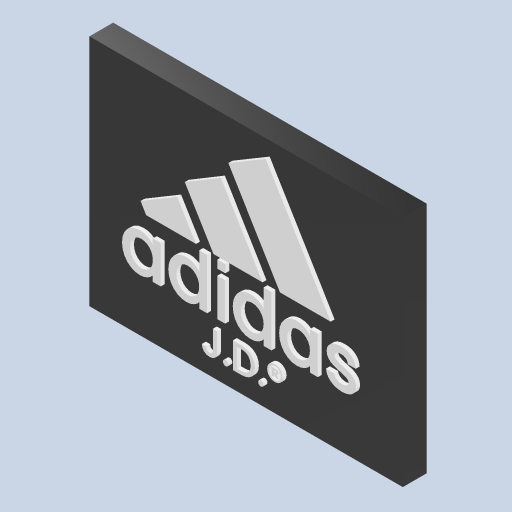
# Autodesk Inventor part: Logo1
Saved by Autodesk Inventor 2023 (Build 270158000, 158)
## iProperties
Created: 2024-02-26
Part Number: Logo1
Material: Generic
Document SubType Name: Modeling
Designer: dsone
Density: 1 g/cm^3
Appearance: Default
Author: dsone
Autodesk Inventor part; units mm, degrees
ref_plane "YZ Plane" through (0, 0, 0) normal (1, 0, 0) x (0, 1, 0)
ref_plane "XZ Plane" through (0, 0, 0) normal (0, 1, 0) x (-1, 0, 0)
ref_plane "XY Plane" through (0, 0, 0) normal (0, 0, 1) x (1, 0, 0)
sketch "Sketch1" plane through (0, 0, 0) normal (0, 0, 1) x (1, 0, 0)
  line L0 (0, 0) -> (240, 0)
  line L1 (240, 0) -> (240, 137)
  line L2 (240, 137) -> (0, 137)
  line L3 (0, 137) -> (0, 0)
  line L4 (0, 0) -> (0, 12)
  line L5 (240, 137) -> (209, 137)
  line L6 (0, 137) -> (10, 137)
  line L7 (0, 137) -> (72, 137)
  line L8 (0, 137) -> (94, 137)
  line L9 (0, 137) -> (158, 137)
  line L10 (0, 137) -> (183, 137)
  line L11 (0, 0) -> (0, 27)
  line L12 (0, 0) -> (0, 43)
  line L13 (0, 0) -> (0, 116)
  line L14 (0, 0) -> (7, 0)
  line L15 (0, 0) -> (70, 0)
  line L16 (0, 0) -> (92, 0)
  line L17 (0, 0) -> (154, 0)
  line L18 (0, 0) -> (176, 0)
  line L19 (7, 0) -> (0, 12)
  line L20 (70, 0) -> (46.1151, 39.5808)
  line L21 (92, 0) -> (55.7734, 60.525)
  line L22 (154, 0) -> (101.369, 87.9322)
  line L23 (176, 0) -> (110.8056, 108.9223)
  line L24 (240, 0) -> (158, 137)
  line L25 (110.8056, 108.9223) -> (158, 137)
  line L26 (0, 12) -> (46.1151, 39.5808)
  line L27 (55.7734, 60.525) -> (101.369, 87.9322)
  line L28 (-19.7944, -2.3315) -> (269.4882, -2.3315) construction
  line L29 (269.4882, -2.3315) -> (269.4882, -75.7518) construction
  line L30 (269.4882, -75.7518) -> (-19.7944, -75.7518) construction
  line L31 (-19.7944, -75.7518) -> (-19.7944, -2.3315) construction
  line L32 (14.2994, -81.6937) -> (242.7128, -81.6937) construction
  line L33 (242.7128, -81.6937) -> (242.7128, -137.0896) construction
  line L34 (242.7128, -137.0896) -> (14.2994, -137.0896) construction
  line L35 (14.2994, -137.0896) -> (14.2994, -81.6937) construction
  spline S0 degree 2 poles (-23.4452, -44.8067) (-23.4452, -37.678) (-17.5046, -26.6137) (-7.2571, -20.4503) (-1.0194, -20.4503) knots 0 0 0 1 2 3 3 3
  spline S1 degree 2 poles (-1.0194, -20.4503) (4.6241, -20.4503) (12.9409, -24.9057) (15.4657, -28.1731) knots 0 0 0 1 2 2 2
  line L36 (15.4657, -28.1731) -> (15.4657, -21.2671)
  line L37 (15.4657, -21.2671) -> (25.4162, -21.2671)
  line L38 (25.4162, -21.2671) -> (25.4162, -68.7919)
  line L39 (25.4162, -68.7919) -> (15.4657, -68.7919)
  line L40 (15.4657, -68.7919) -> (15.4657, -61.7374)
  spline S2 degree 2 poles (15.4657, -61.7374) (12.9409, -65.079) (4.3271, -69.5344) (-1.168, -69.5344) knots 0 0 0 1 2 2 2
  spline S3 degree 2 poles (-1.168, -69.5344) (-7.3313, -69.5344) (-17.5046, -63.2968) (-23.4452, -51.9354) (-23.4452, -44.8067) knots 0 0 0 1 2 3 3 3
  spline S4 degree 2 poles (15.4657, -44.9552) (15.4657, -40.0542) (11.3815, -32.777) (4.8469, -28.9899) (1.0598, -28.9899) knots 0 0 0 1 2 3 3 3
  spline S5 degree 2 poles (1.0598, -28.9899) (-2.7274, -28.9899) (-9.262, -32.7028) (-13.3462, -39.9057) (-13.3462, -44.8067) knots 0 0 0 1 2 3 3 3
  spline S6 degree 2 poles (-13.3462, -44.8067) (-13.3462, -49.7077) (-9.262, -57.1335) (-2.6531, -60.9948) (1.0598, -60.9948) knots 0 0 0 1 2 3 3 3
  spline S7 degree 2 poles (1.0598, -60.9948) (4.8469, -60.9948) (11.3815, -57.2077) (15.4657, -49.9305) (15.4657, -44.9552) knots 0 0 0 1 2 3 3 3
  spline S8 degree 2 poles (35.0697, -44.8067) (35.0697, -37.678) (41.0103, -26.6137) (51.2578, -20.4503) (57.5697, -20.4503) knots 0 0 0 1 2 3 3 3
  spline S9 degree 2 poles (57.5697, -20.4503) (62.2479, -20.4503) (71.3073, -24.5344) (73.9806, -27.876) knots 0 0 0 1 2 2 2
  line L41 (73.9806, -27.876) -> (73.9806, -4.9305)
  line L42 (73.9806, -4.9305) -> (83.931, -4.9305)
  line L43 (83.931, -4.9305) -> (83.931, -68.7919)
  line L44 (83.931, -68.7919) -> (73.9806, -68.7919)
  line L45 (73.9806, -68.7919) -> (73.9806, -61.6632)
  spline S10 degree 2 poles (73.9806, -61.6632) (71.6043, -65.079) (62.9905, -69.5344) (57.4954, -69.5344) knots 0 0 0 1 2 2 2
  spline S11 degree 2 poles (57.4954, -69.5344) (51.2578, -69.5344) (41.0103, -63.2968) (35.0697, -51.9354) (35.0697, -44.8067) knots 0 0 0 1 2 3 3 3
  spline S12 degree 2 poles (73.9806, -44.9552) (73.9806, -40.0542) (69.8964, -32.777) (63.3617, -28.9899) (59.5746, -28.9899) knots 0 0 0 1 2 3 3 3
  spline S13 degree 2 poles (59.5746, -28.9899) (55.7875, -28.9899) (49.2528, -32.7028) (45.1687, -39.9057) (45.1687, -44.8067) knots 0 0 0 1 2 3 3 3
  spline S14 degree 2 poles (45.1687, -44.8067) (45.1687, -49.7077) (49.2528, -57.1335) (55.8617, -60.9948) (59.5746, -60.9948) knots 0 0 0 1 2 3 3 3
  spline S15 degree 2 poles (59.5746, -60.9948) (63.3617, -60.9948) (69.8964, -57.2077) (73.9806, -49.9305) (73.9806, -44.9552) knots 0 0 0 1 2 3 3 3
  line L46 (106.7281, -21.2671) -> (106.7281, -68.7919)
  line L47 (106.7281, -68.7919) -> (96.8518, -68.7919)
  line L48 (96.8518, -68.7919) -> (96.8518, -21.2671)
  line L49 (96.8518, -21.2671) -> (106.7281, -21.2671)
  spline S16 degree 2 poles (101.9013, -14.9552) (99.2281, -14.9552) (95.5895, -11.3166) (95.5895, -8.6434) knots 0 0 0 1 2 2 2
  spline S17 degree 2 poles (95.5895, -8.6434) (95.5895, -5.9701) (99.2281, -2.3315) (101.9013, -2.3315) knots 0 0 0 1 2 2 2
  spline S18 degree 2 poles (101.9013, -2.3315) (104.4261, -2.3315) (108.0647, -5.9701) (108.0647, -8.6434) knots 0 0 0 1 2 2 2
  spline S19 degree 2 poles (108.0647, -8.6434) (108.0647, -11.3166) (104.4261, -14.9552) (101.9013, -14.9552) knots 0 0 0 1 2 2 2
  spline S20 degree 2 poles (116.3815, -44.8067) (116.3815, -37.678) (122.3221, -26.6137) (132.5697, -20.4503) (138.8815, -20.4503) knots 0 0 0 1 2 3 3 3
  spline S21 degree 2 poles (138.8815, -20.4503) (143.5598, -20.4503) (152.6192, -24.5344) (155.2924, -27.876) knots 0 0 0 1 2 2 2
  line L50 (155.2924, -27.876) -> (155.2924, -4.9305)
  line L51 (155.2924, -4.9305) -> (165.2429, -4.9305)
  line L52 (165.2429, -4.9305) -> (165.2429, -68.7919)
  line L53 (165.2429, -68.7919) -> (155.2924, -68.7919)
  line L54 (155.2924, -68.7919) -> (155.2924, -61.6632)
  spline S22 degree 2 poles (155.2924, -61.6632) (152.9162, -65.079) (144.3023, -69.5344) (138.8073, -69.5344) knots 0 0 0 1 2 2 2
  spline S23 degree 2 poles (138.8073, -69.5344) (132.5697, -69.5344) (122.3221, -63.2968) (116.3815, -51.9354) (116.3815, -44.8067) knots 0 0 0 1 2 3 3 3
  spline S24 degree 2 poles (155.2924, -44.9552) (155.2924, -40.0542) (151.2083, -32.777) (144.6736, -28.9899) (140.8865, -28.9899) knots 0 0 0 1 2 3 3 3
  spline S25 degree 2 poles (140.8865, -28.9899) (137.0994, -28.9899) (130.5647, -32.7028) (126.4806, -39.9057) (126.4806, -44.8067) knots 0 0 0 1 2 3 3 3
  spline S26 degree 2 poles (126.4806, -44.8067) (126.4806, -49.7077) (130.5647, -57.1335) (137.1736, -60.9948) (140.8865, -60.9948) knots 0 0 0 1 2 3 3 3
  spline S27 degree 2 poles (140.8865, -60.9948) (144.6736, -60.9948) (151.2083, -57.2077) (155.2924, -49.9305) (155.2924, -44.9552) knots 0 0 0 1 2 3 3 3
  spline S28 degree 2 poles (174.8964, -44.8067) (174.8964, -37.678) (180.837, -26.6137) (191.0845, -20.4503) (197.3221, -20.4503) knots 0 0 0 1 2 3 3 3
  spline S29 degree 2 poles (197.3221, -20.4503) (202.9657, -20.4503) (211.2825, -24.9057) (213.8073, -28.1731) knots 0 0 0 1 2 2 2
  line L55 (213.8073, -28.1731) -> (213.8073, -21.2671)
  line L56 (213.8073, -21.2671) -> (223.7578, -21.2671)
  line L57 (223.7578, -21.2671) -> (223.7578, -68.7919)
  line L58 (223.7578, -68.7919) -> (213.8073, -68.7919)
  line L59 (213.8073, -68.7919) -> (213.8073, -61.7374)
  spline S30 degree 2 poles (213.8073, -61.7374) (211.2825, -65.079) (202.6687, -69.5344) (197.1736, -69.5344) knots 0 0 0 1 2 2 2
  spline S31 degree 2 poles (197.1736, -69.5344) (191.0103, -69.5344) (180.837, -63.2968) (174.8964, -51.9354) (174.8964, -44.8067) knots 0 0 0 1 2 3 3 3
  spline S32 degree 2 poles (213.8073, -44.9552) (213.8073, -40.0542) (209.7231, -32.777) (203.1885, -28.9899) (199.4013, -28.9899) knots 0 0 0 1 2 3 3 3
  spline S33 degree 2 poles (199.4013, -28.9899) (195.6142, -28.9899) (189.0796, -32.7028) (184.9954, -39.9057) (184.9954, -44.8067) knots 0 0 0 1 2 3 3 3
  spline S34 degree 2 poles (184.9954, -44.8067) (184.9954, -49.7077) (189.0796, -57.1335) (195.6885, -60.9948) (199.4013, -60.9948) knots 0 0 0 1 2 3 3 3
  spline S35 degree 2 poles (199.4013, -60.9948) (203.1885, -60.9948) (209.7231, -57.2077) (213.8073, -49.9305) (213.8073, -44.9552) knots 0 0 0 1 2 3 3 3
  spline S36 degree 2 poles (253.9806, -69.5344) (248.337, -69.5344) (239.4261, -65.5245) (234.3023, -58.5443) (234.0796, -54.2374) knots 0 0 0 1 2 3 3 3
  line L60 (234.0796, -54.2374) -> (244.2528, -54.2374)
  spline S37 degree 2 poles (244.2528, -54.2374) (244.5499, -57.2077) (249.8221, -61.2919) (253.7578, -61.2919) knots 0 0 0 1 2 2 2
  spline S38 degree 2 poles (253.7578, -61.2919) (257.9162, -61.2919) (262.5202, -58.0988) (262.5202, -55.5741) knots 0 0 0 1 2 2 2
  spline S39 degree 2 poles (262.5202, -55.5741) (262.5202, -52.9008) (257.3964, -50.3018) (251.9013, -48.7424) knots 0 0 0 1 2 2 2
  spline S40 degree 2 poles (251.9013, -48.7424) (246.5548, -47.3315) (239.7974, -44.5097) (234.8964, -38.8661) (234.8964, -34.1879) knots 0 0 0 1 2 3 3 3
  spline S41 degree 2 poles (234.8964, -34.1879) (234.8964, -30.4008) (239.3518, -24.0889) (247.7429, -20.4503) (253.1637, -20.4503) knots 0 0 0 1 2 3 3 3
  spline S42 degree 2 poles (253.1637, -20.4503) (261.2578, -20.4503) (271.2083, -28.6929) (271.5796, -35.7473) knots 0 0 0 1 2 2 2
  line L61 (271.5796, -35.7473) -> (261.7033, -35.7473)
  spline S43 degree 2 poles (261.7033, -35.7473) (261.4806, -32.5542) (256.8023, -28.7671) (252.7924, -28.7671) knots 0 0 0 1 2 2 2
  spline S44 degree 2 poles (252.7924, -28.7671) (248.931, -28.7671) (244.7726, -31.6632) (244.7726, -34.1137) knots 0 0 0 1 2 2 2
  spline S45 degree 2 poles (244.7726, -34.1137) (244.7726, -35.9701) (247.5944, -38.5691) (251.5301, -40.0542) (255.3914, -41.1681) knots 0 0 0 1 2 3 3 3
  spline S46 degree 2 poles (255.3914, -41.1681) (260.5895, -42.579) (267.2726, -45.4008) (272.0994, -50.8958) (272.1736, -55.4998) knots 0 0 0 1 2 3 3 3
  spline S47 degree 2 poles (272.1736, -55.4998) (272.1736, -59.584) (267.6439, -65.9701) (259.4756, -69.5344) (253.9806, -69.5344) knots 0 0 0 1 2 3 3 3
  line L62 (96.6197, -82.1362) -> (96.6197, -105.5933)
  spline S48 degree 2 poles (96.6197, -105.5933) (96.6197, -109.9387) (91.3087, -114.9681) (87.0035, -114.9681) knots 0 0 0 1 2 2 2
  spline S49 degree 2 poles (87.0035, -114.9681) (82.6984, -114.9681) (77.4276, -109.9387) (77.4276, -105.5933) knots 0 0 0 1 2 2 2
  line L63 (77.4276, -105.5933) -> (82.8191, -105.5933)
  spline S50 degree 2 poles (82.8191, -105.5933) (82.8593, -107.7258) (84.9515, -110.2606) (87.0035, -110.2606) knots 0 0 0 1 2 2 2
  spline S51 degree 2 poles (87.0035, -110.2606) (89.0555, -110.2606) (91.2282, -107.6856) (91.2282, -105.5933) knots 0 0 0 1 2 2 2
  line L64 (91.2282, -105.5933) -> (91.2282, -82.1362)
  line L65 (91.2282, -82.1362) -> (96.6197, -82.1362)
  spline S52 degree 2 poles (107.443, -114.9681) (105.9945, -114.9681) (104.023, -112.9966) (104.023, -111.5481) knots 0 0 0 1 2 2 2
  spline S53 degree 2 poles (104.023, -111.5481) (104.023, -110.0997) (105.9945, -108.1281) (107.443, -108.1281) knots 0 0 0 1 2 2 2
  spline S54 degree 2 poles (107.443, -108.1281) (108.811, -108.1281) (110.7825, -110.0997) (110.7825, -111.5481) knots 0 0 0 1 2 2 2
  spline S55 degree 2 poles (110.7825, -111.5481) (110.7825, -112.9966) (108.811, -114.9681) (107.443, -114.9681) knots 0 0 0 1 2 2 2
  spline S56 degree 2 poles (127.1582, -82.1362) (132.3485, -82.1362) (140.1542, -86.1195) (144.4191, -93.563) (144.4191, -98.5119) knots 0 0 0 1 2 3 3 3
  spline S57 degree 2 poles (144.4191, -98.5119) (144.4191, -103.4609) (140.1542, -110.7837) (132.3485, -114.6462) (127.1582, -114.6462) knots 0 0 0 1 2 3 3 3
  line L66 (127.1582, -114.6462) -> (116.5361, -114.6462)
  line L67 (116.5361, -114.6462) -> (116.5361, -82.1362)
  line L68 (116.5361, -82.1362) -> (127.1582, -82.1362)
  spline S58 degree 2 poles (127.1582, -110.3008) (132.8716, -110.3008) (138.9471, -104.1449) (138.9471, -98.5119) knots 0 0 0 1 2 2 2
  spline S59 degree 2 poles (138.9471, -98.5119) (138.9471, -92.879) (132.8716, -86.4816) (127.1582, -86.4816) knots 0 0 0 1 2 2 2
  line L69 (127.1582, -86.4816) -> (121.8874, -86.4816)
  line L70 (121.8874, -86.4816) -> (121.8874, -110.3008)
  line L71 (121.8874, -110.3008) -> (127.1582, -110.3008)
  spline S60 degree 2 poles (151.8626, -114.9681) (150.4141, -114.9681) (148.4426, -112.9966) (148.4426, -111.5481) knots 0 0 0 1 2 2 2
  spline S61 degree 2 poles (148.4426, -111.5481) (148.4426, -110.0997) (150.4141, -108.1281) (151.8626, -108.1281) knots 0 0 0 1 2 2 2
  spline S62 degree 2 poles (151.8626, -108.1281) (153.2306, -108.1281) (155.2021, -110.0997) (155.2021, -111.5481) knots 0 0 0 1 2 2 2
  spline S63 degree 2 poles (155.2021, -111.5481) (155.2021, -112.9966) (153.2306, -114.9681) (151.8626, -114.9681) knots 0 0 0 1 2 2 2
  spline S64 degree 2 poles (169.5661, -81.6937) (172.3825, -81.6937) (176.8084, -84.2285) (179.303, -88.6543) (179.303, -91.4708) knots 0 0 0 1 2 3 3 3
  spline S65 degree 2 poles (179.303, -91.4708) (179.303, -94.247) (176.8084, -98.7131) (172.3825, -101.2077) (169.5661, -101.2077) knots 0 0 0 1 2 3 3 3
  spline S66 degree 2 poles (169.5661, -101.2077) (166.7496, -101.2077) (162.3237, -98.7131) (159.7889, -94.247) (159.7889, -91.4708) knots 0 0 0 1 2 3 3 3
  spline S67 degree 2 poles (159.7889, -91.4708) (159.7889, -88.6543) (162.3237, -84.2285) (166.7496, -81.6937) (169.5661, -81.6937) knots 0 0 0 1 2 3 3 3
  spline S68 degree 2 poles (169.5661, -99.0752) (172.9458, -99.0752) (177.0096, -94.8505) (177.0096, -91.4708) knots 0 0 0 1 2 2 2
  spline S69 degree 2 poles (177.0096, -91.4708) (177.0096, -88.0508) (172.9458, -83.8261) (169.5661, -83.8261) knots 0 0 0 1 2 2 2
  spline S70 degree 2 poles (169.5661, -83.8261) (166.1461, -83.8261) (162.1226, -88.0508) (162.1226, -91.4708) knots 0 0 0 1 2 2 2
  spline S71 degree 2 poles (162.1226, -91.4708) (162.1226, -94.8505) (166.1461, -99.0752) (169.5661, -99.0752) knots 0 0 0 1 2 2 2
  spline S72 degree 2 poles (173.8712, -89.5797) (173.8712, -90.6259) (172.8251, -92.1548) (171.9399, -92.5169) knots 0 0 0 1 2 2 2
  line L72 (171.9399, -92.5169) -> (174.4345, -96.3795)
  line L73 (174.4345, -96.3795) -> (170.8938, -96.3795)
  line L74 (170.8938, -96.3795) -> (168.8016, -92.879)
  line L75 (168.8016, -92.879) -> (168.4797, -92.879)
  line L76 (168.4797, -92.879) -> (168.4797, -96.3795)
  line L77 (168.4797, -96.3795) -> (165.5425, -96.3795)
  line L78 (165.5425, -96.3795) -> (165.5425, -86.3207)
  line L79 (165.5425, -86.3207) -> (170.2501, -86.3207)
  spline S73 degree 2 poles (170.2501, -86.3207) (171.8997, -86.3207) (173.8712, -88.1313) (173.8712, -89.5797) knots 0 0 0 1 2 2 2
  line L80 (168.4797, -90.4649) -> (170.0891, -90.4649)
  spline S74 degree 2 poles (170.0891, -90.4649) (170.4512, -90.4649) (170.9743, -90.0626) (170.9743, -89.6602) knots 0 0 0 1 2 2 2
  spline S75 degree 2 poles (170.9743, -89.6602) (170.9743, -89.2981) (170.4512, -88.936) (170.0891, -88.936) knots 0 0 0 1 2 2 2
  line L81 (170.0891, -88.936) -> (168.4797, -88.936)
  line L82 (168.4797, -88.936) -> (168.4797, -90.4649)
  dimension "d0" = 240
  dimension "d1" = 137
  dimension "d2" = 12
  dimension "d3" = 31
  dimension "d4" = 10
  dimension "d5" = 72
  dimension "d6" = 94
  dimension "d7" = 158
  dimension "d8" = 183
  dimension "d9" = 27
  dimension "d10" = 43
  dimension "d11" = 116
  dimension "d12" = 7
  dimension "d13" = 70
  dimension "d14" = 92
  dimension "d15" = 154
  dimension "d16" = 176
  constraints: 56 end point, 15 point on line, 2 horizontal, 2 perpendicular, 4 other
  measures "d0" distance of L0.start L0.end
  measures "d1" distance of L0.end L1.end
  measures "d2" distance of L0.start L4.end
  measures "d3" distance of L1.end L5.end
  measures "d4" distance of L2.end L6.end
  measures "d5" distance of L2.end L7.end
  measures "d6" distance of L2.end L8.end
  measures "d7" distance of L2.end L9.end
  measures "d8" distance of L2.end L10.end
  measures "d9" distance of L0.start L11.end
  measures "d10" distance of L0.start L12.end
  measures "d11" distance of L0.start L13.end
  measures "d12" distance of L0.start L14.end
  measures "d13" distance of L0.start L15.end
  measures "d14" distance of L0.start L16.end
  measures "d15" distance of L0.start L17.end
  measures "d16" distance of L0.start L18.end
extrude "Extrusion1" add sketch "Sketch1" along normal blind 5 contours S0 S1 L36 L37 L38 L39 L40 S2 S3 | S8 S9 L41 L42 L43 L44 L45 S10 S11 | L46 L47 L48 L49 | S16 S17 S18 S19 | S20 S21 L50 L51 L52 L53 L54 S22 S23 | S28 S29 L55 L56 L57 L58 L59 S30 S31 | S36 L60 S37 S38 S39 S40 S41 S42 L61 S43 S44 S45 S46 S47
extrude "Extrusion2" add sketch "Sketch1" along normal blind 5 contours L21 L27 L22 L0
extrude "Extrusion3" add sketch "Sketch1" along normal blind 5 contours L23 L25 L24 L0
extrude "Extrusion4" add sketch "Sketch1" along normal blind 5 contours L19 L26 L20 L0
sketch "Sketch2" plane through (0, 0, 5) normal (0, 0, 1) x (1, 0, 0)
  spline S0 degree 2 poles (95.5895, -8.6434) (95.5895, -11.3166) (99.2281, -14.9552) (101.9013, -14.9552) knots 0 0 0 0.5 1 1 1 projected
  spline S1 degree 2 poles (101.9013, -14.9552) (104.4261, -14.9552) (108.0647, -11.3166) (108.0647, -8.6434) knots 0 0 0 0.5 1 1 1 projected
  spline S2 degree 2 poles (108.0647, -8.6434) (108.0647, -5.9701) (104.4261, -2.3315) (101.9013, -2.3315) knots 0 0 0 0.5 1 1 1 projected
  spline S3 degree 2 poles (101.9013, -2.3315) (99.2281, -2.3315) (95.5895, -5.9701) (95.5895, -8.6434) knots 0 0 0 0.5 1 1 1 projected
  line L0 (96.9113, -3.6534) -> (106.8913, -3.6534)
  line L1 (106.8913, -3.6534) -> (106.8913, -13.6334)
  line L2 (106.8913, -13.6334) -> (96.9113, -13.6334)
  line L3 (96.9113, -13.6334) -> (96.9113, -3.6534)
  line L4 (96.9113, -3.6534) -> (106.8913, -13.6334) construction
  line L5 (106.8913, -3.6534) -> (96.9113, -13.6334) construction
  point P0 (0, 0)
  point P1 (101.9013, -8.6434)
  point P2 (96.9113, -12.5803)
  point P3 (96.9113, -4.7064)
  point P4 (106.8913, -4.9004)
  point P5 (106.8913, -12.3863)
  point P6 (105.693, -13.6334)
  point P7 (97.9644, -13.6334)
  point P8 (97.9644, -3.6534)
  point P9 (105.693, -3.6534)
  dimension "d25" = 9.98
  dimension "d26" = 9.98
  constraints: 12 end point, 2 midpoint, 2 parallel, 1 horizontal, 1 perpendicular, 4 other
  measures "d25" distance of L1.end L2.end
  measures "d26" distance of L0.end L1.end
extrude "Extrusion5" cut sketch "Sketch2" against normal blind 5 contours S3 L3 S0
extrude "Extrusion6" cut sketch "Sketch2" against normal blind 5 contours L1 S2 S1
extrude "Extrusion7" cut sketch "Sketch2" against normal blind 5 contours L2 S1 S0
extrude "Extrusion8" cut sketch "Sketch2" against normal blind 5 contours S3 S2 L0
extrude "Extrusion9" add sketch "Sketch2" against normal blind 5 contours S0 L2 L3 | L3 L0 S3 | S1 L1 L2 | L0 L1 S2
sketch "Sketch4" plane through (0, 0, 0) normal (0, 0, -1) x (-1, 0, 0)
  line L0 (69.5948, -140.3243) -> (-326.0365, -140.3243)
  line L1 (-326.0365, -140.3243) -> (-326.0365, 154.6971)
  line L2 (-326.0365, 154.6971) -> (69.5948, 154.6971)
  line L3 (69.5948, 154.6971) -> (69.5948, -140.3243)
  point P0 (0, 0)
  constraints: 8 end point, 2 parallel, 1 horizontal, 1 perpendicular
extrude "Extrusion11" add sketch "Sketch1" along normal blind 5 contours L62 S48 S49 L63 S50 S51 L64 L65 | S52 S53 S54 S55 | S56 S57 L66 L67 L68 | S60 S61 S62 S63 | S64 S65 S66 S67 | S72 L72 L73 L74 L75 L76 L77 L78 L79 S73
extrude "Extrusion12" add sketch "Sketch4" along normal blind 30
body "Solid1"
